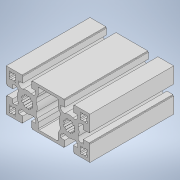
# Autodesk Inventor part: perfil-aluminio-0002-001
Saved by Autodesk Inventor 2020.1 (Build 241239000, 239)
## iProperties
Created: 2024-04-13
Part Number: perfil-aluminio-0002-001
Material: Generic
Document SubType Name: Modeling
Designer: MiguelBarbosa
Density: 1 g/cm^3
Appearance: Default
Author: MiguelBarbosa
Autodesk Inventor part; units mm, degrees
ref_plane "YZ Plane" through (0, 0, 0) normal (1, 0, 0) x (0, 1, 0)
ref_plane "XZ Plane" through (0, 0, 0) normal (0, 1, 0) x (-1, 0, 0)
ref_plane "XY Plane" through (0, 0, 0) normal (0, 0, 1) x (1, 0, 0)
sketch "Sketch1" plane through (0, 0, 0) normal (0, 0, 1) x (1, 0, 0)
  circle A0 centre (-25, 0) radius 6
  line L0 (0, 0) -> (-25, 0) construction
  circle A1 centre (-25, 0) radius 12
  line L1 (-45.9, 14.1) -> (-39.1, 14.1) construction
  line L2 (-39.1, 14.1) -> (-39.1, 20.9) construction
  line L3 (-39.1, 20.9) -> (-45.9, 20.9) construction
  line L4 (-45.9, 20.9) -> (-45.9, 14.1) construction
  line L5 (-45.9, 14.1) -> (-39.1, 20.9) construction
  line L6 (-39.1, 14.1) -> (-45.9, 20.9) construction
  line L7 (-46.5, 13.5) -> (-38.5, 13.5) construction
  line L8 (-38.5, 13.5) -> (-38.5, 21.5) construction
  line L9 (-38.5, 21.5) -> (-46.5, 21.5) construction
  line L10 (-46.5, 21.5) -> (-46.5, 13.5) construction
  line L11 (-46.5, 13.5) -> (-38.5, 21.5) construction
  line L12 (-38.5, 13.5) -> (-46.5, 21.5) construction
  line L13 (-44, 20.9) -> (-41, 20.9)
  line L14 (-44, 20.9) -> (-44, 21.5)
  line L15 (-44, 21.5) -> (-46.5, 21.5)
  line L16 (-41, 20.9) -> (-41, 21.5)
  line L17 (-41, 21.5) -> (-38.5, 21.5)
  line L18 (-46.5, 21.5) -> (-46.5, 19)
  line L19 (-46.5, 19) -> (-45.9, 19)
  line L20 (-45.9, 19) -> (-45.9, 16)
  line L21 (-45.9, 16) -> (-46.5, 16)
  line L22 (-46.5, 16) -> (-46.5, 13.5)
  line L23 (-46.5, 13.5) -> (-44, 13.5)
  line L24 (-44, 13.5) -> (-44, 14.1)
  line L25 (-44, 14.1) -> (-41, 14.1)
  line L26 (-41, 14.1) -> (-41, 13.5)
  line L27 (-41, 13.5) -> (-38.5, 13.5)
  line L28 (-38.5, 13.5) -> (-38.5, 16)
  line L29 (-38.5, 16) -> (-39.1, 16)
  line L30 (-39.1, 16) -> (-39.1, 19)
  line L31 (-39.1, 19) -> (-38.5, 19)
  line L32 (-38.5, 19) -> (-38.5, 21.5)
  line L33 (-50, 25) -> (-50, 5.1) construction
  line L34 (-50, 25) -> (-30.1, 25) construction
  line L35 (-50, 5.1) -> (-49, 5.1) construction
  line L36 (-49, 5.1) -> (-49, 6.1)
  line L37 (-49, 6.1) -> (-50, 6.1)
  line L38 (-50, 6.1) -> (-50, 5.1) construction
  line L39 (-50, 5.1) -> (-49, 6.1) construction
  line L40 (-49, 5.1) -> (-50, 6.1) construction
  line L41 (-50, 6.1) -> (-50, 25)
  line L42 (-31.1, 24) -> (-30.1, 24)
  line L43 (-30.1, 24) -> (-30.1, 25) construction
  line L44 (-30.1, 25) -> (-31.1, 25) construction
  line L45 (-31.1, 25) -> (-31.1, 24)
  line L46 (-31.1, 24) -> (-30.1, 25) construction
  line L47 (-30.1, 24) -> (-31.1, 25) construction
  line L48 (-50, 25) -> (-31.1, 25)
  line L49 (-30.1, 24) -> (-30.1, 17)
  line L50 (-30.1, 17) -> (-35.1, 17)
  line L51 (-35.1, 17) -> (-35.1, 12) construction
  line L52 (-35.1, 12) -> (-25, 12) construction
  arc A2 (-35.1, 14.5) -> (-29.7776, 11.0079) centre (-31.2932, 14.5) ccw
  line L53 (-35.1, 17) -> (-35.1, 14.5)
  line L54 (-49, 5.1) -> (-42, 5.1)
  line L55 (-42, 5.1) -> (-42, 10.1)
  line L56 (-42, 10.1) -> (-39.5, 10.1)
  arc A3 (-36.0079, 4.7776) -> (-39.5, 10.1) centre (-39.5, 6.2932) ccw
  arc A4 (-20.2224, 11.0079) -> (-14.9, 14.5) centre (-18.7068, 14.5) ccw
  line L57 (-14.9, 14.5) -> (-14.9, 17)
  line L58 (-14.9, 17) -> (-19.9, 17)
  line L59 (-19.9, 17) -> (-19.9, 24)
  line L60 (-19.9, 24) -> (-18.9, 24)
  line L61 (-18.9, 24) -> (-18.9, 25)
  line L62 (-18.9, 25) -> (-19.9, 25) construction
  line L63 (-19.9, 25) -> (-19.9, 24) construction
  line L64 (-19.9, 24) -> (-18.9, 25) construction
  line L65 (-18.9, 24) -> (-19.9, 25) construction
  line L66 (-18.9, 25) -> (0, 25)
  line L67 (0, 22) -> (-11.9, 22) construction
  line L68 (-11.9, 22) -> (-11.9, 14.5) construction
  arc A5 (-13.1902, 10.8149) -> (-13.9921, 4.7776) centre (-8.5727, 7.1297) ccw
  arc A6 (-13.1902, 10.8149) -> (-11.9, 14.5) centre (-17.8078, 14.5) ccw
  line L69 (0, 22) -> (0, 25)
  arc A7 (-10.9, 22) -> (-11.9, 21) centre (-10.9, 21) ccw
  line L70 (-11.9, 21) -> (-11.9, 14.5)
  line L71 (-10.9, 22) -> (0, 22)
  point P0 (-42.5, 17.5)
  point P1 (-42.5, 17.5)
  point P2 (-42.5, 17.5)
  point P3 (-42.5, 20.9)
  point P4 (-49.5, 5.6)
  point P5 (-30.6, 24.5)
  point P6 (-19.4, 24.5)
  dimension "d0" = 25
  dimension "d1" = 12
  dimension "d2" = 24
  dimension "d16" = 17.5
  dimension "d17" = 42.5
  dimension "d18" = 6.8
  dimension "d19" = 8
  dimension "d20" = 3
  dimension "d21" = 5.1
  dimension "d22" = 25
  dimension "d23" = 50
  dimension "d24" = 1
  dimension "d25" = 7
  dimension "d26" = 5
  dimension "d27" = 5
  dimension "d30" = 3
  dimension "d31" = 3
  dimension "d34" = 1
  constraints: 144 end point, 20 equal length, 16 horizontal, 16 point on circle, 15 midpoint, 14 point on line, 12 tangent, 12 vertical, 11 perpendicular, 10 parallel, 9 collinear, 8 centre point, 3 coincident, 3 horizontal alignment, 3 vertical alignment, 2 equal radius
  measures "d0" distance of L0.start L0.end
  measures "d1" diameter of A0
  measures "d2" diameter of A1
  measures "d16" horizontal distance of A0.centre point (-42.5, 17.5)
  measures "d17" horizontal distance of point (0, 0) point (-42.5, 17.5)
  measures "d18" distance of L2.end L3.end
  measures "d19" distance of L8.end L9.end
  measures "d20" distance of L13.start L13.end
  measures "d21" vertical distance of point (0, 0) L33.end
  measures "d22" vertical distance of point (0, 0) L33.start
  measures "d23" horizontal distance of point (0, 0) L33.start
  measures "d24" distance of L36.end L37.end
  measures "d25" distance of L42.end L49.end
  measures "d26" distance of L49.end L50.end
  measures "d27" distance of L50.end L51.end
  measures "d30" distance between parallel lines of L66 L67
  measures "d31" distance between parallel lines of L57 L68
  measures "d34" radius of A7
extrude "Extrusion1" add sketch "Sketch1" along normal mid plane 100 contours A1
sketch "Sketch2" plane through (-25, 0, 50) normal (0, 0, 1) x (1, 0, 0)
  circle A0 centre (0, 0) radius 6 construction
  line L0 (0, 0) -> (1.3656, 6.8655) construction
  circle A1 centre (0, 0) radius 7 construction
  line L1 (0, 0) -> (-1.3656, 6.8655) construction
  line L2 (0, 0) -> (0, 7) construction
  line L3 (0, 0) -> (-3.889, 5.8203) construction
  arc A2 (-1.1705, 5.8847) -> (-3.3334, 4.9888) centre (0, 0) ccw
  line L4 (-3.3334, 4.9888) -> (-3.889, 5.8203)
  line L5 (-1.1705, 5.8847) -> (-1.3656, 6.8655)
  arc A3 (-1.3656, 6.8655) -> (-3.889, 5.8203) centre (0, 0) ccw
  point P0 (25, 0)
  point P1 (-2.6788, 6.4672)
  dimension "d5" = 14
  dimension "d6" = 22.5
  dimension "d7" = 22.5
  constraints: 12 end point, 12 point on circle, 3 centre point, 2 collinear, 2 point on line, 1 coincident, 1 concentric, 1 vertical, 1 other
  measures "d5" diameter of A1
  measures "d6" angle of L0 L1
  measures "d7" angle of L1 L3
extrude "Extrusion2" cut sketch "Sketch2" against normal through all
pattern_circular "Circular Pattern2" count 8 over 360 about axis through (-25, 0, 0) along (0, 0, 1) of "Extrusion2"
extrude "Extrusion3" add sketch "Sketch1" along normal mid plane 100 contours A3 L56 L55 L54 L36 L37 L41 L48 L45 L42 L49 L50 L53 A2 A1
mirror "Mirror1" about plane through (0, 0, 0) normal (0, 1, 0) of "Extrusion3"
extrude "Extrusion4" add sketch "Sketch1" along normal mid plane 100 contours A1 A4 L57 L58 L59 L60 L61 L66 L69 L71 A7 L70 A6 A5
mirror "Mirror2" about plane through (0, 0, 0) normal (0, 1, 0) of "Extrusion4"
mirror "Mirror3" about plane through (0, 0, 0) normal (1, 0, 0) of "Extrusion1", "Extrusion2", "Circular Pattern2", "Extrusion3", "Mirror1", "Extrusion4", "Mirror2"
equation "\"d31\" = d30"
equation "\"d7\" = d6"
body "Solid1"
